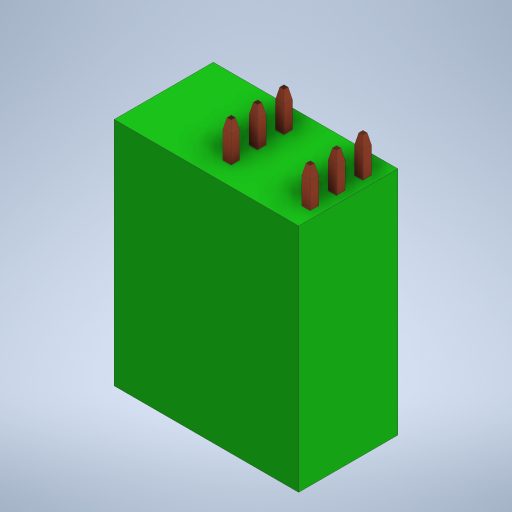
# Autodesk Inventor part: DB2ERH-2.5-2x3
Saved by Autodesk Inventor 2024 (Build 280153000, 153)
## iProperties
Created: 2023-05-22
Part Number: DB2ERH-2.5-2x3
Material: Generic
Document SubType Name: Modeling
Designer: torba
Density: 1 g/cm^3
Appearance: Default
Author: torba
Autodesk Inventor part; units mm, degrees
ref_plane "YZ Plane" through (0, 0, 0) normal (1, 0, 0) x (0, 1, 0)
ref_plane "XZ Plane" through (0, 0, 0) normal (0, 1, 0) x (-1, 0, 0)
ref_plane "XY Plane" through (0, 0, 0) normal (0, 0, 1) x (1, 0, 0)
sketch "Sketch1" plane through (0, 0, 0) normal (0, 1, 0) x (-1, 0, 0)
  line L0 (-0.4, 0.4) -> (0.4, 0.4)
  line L1 (0.4, 0.4) -> (0.4, -0.4)
  line L2 (0.4, -0.4) -> (-0.4, -0.4)
  line L3 (-0.4, -0.4) -> (-0.4, 0.4)
  line L4 (-0.4, 0.4) -> (0.4, -0.4) construction
  line L5 (0.4, 0.4) -> (-0.4, -0.4) construction
  line L6 (-0.4, -2.1) -> (0.4, -2.1)
  line L7 (0.4, -2.1) -> (0.4, -2.9)
  line L8 (0.4, -2.9) -> (-0.4, -2.9)
  line L9 (-0.4, -2.9) -> (-0.4, -2.1)
  line L10 (-0.4, -2.1) -> (0.4, -2.9) construction
  line L11 (0.4, -2.1) -> (-0.4, -2.9) construction
  line L12 (-0.4, -4.6) -> (0.4, -4.6)
  line L13 (0.4, -4.6) -> (0.4, -5.4)
  line L14 (0.4, -5.4) -> (-0.4, -5.4)
  line L15 (-0.4, -5.4) -> (-0.4, -4.6)
  line L16 (-0.4, -4.6) -> (0.4, -5.4) construction
  line L17 (0.4, -4.6) -> (-0.4, -5.4) construction
  line L18 (-7.9, 0.4) -> (-7.1, 0.4)
  line L19 (-7.1, 0.4) -> (-7.1, -0.4)
  line L20 (-7.1, -0.4) -> (-7.9, -0.4)
  line L21 (-7.9, -0.4) -> (-7.9, 0.4)
  line L22 (-7.9, 0.4) -> (-7.1, -0.4) construction
  line L23 (-7.1, 0.4) -> (-7.9, -0.4) construction
  line L24 (-7.9, -2.1) -> (-7.1, -2.1)
  line L25 (-7.1, -2.1) -> (-7.1, -2.9)
  line L26 (-7.1, -2.9) -> (-7.9, -2.9)
  line L27 (-7.9, -2.9) -> (-7.9, -2.1)
  line L28 (-7.9, -2.1) -> (-7.1, -2.9) construction
  line L29 (-7.1, -2.1) -> (-7.9, -2.9) construction
  line L30 (-7.9, -4.6) -> (-7.1, -4.6)
  line L31 (-7.1, -4.6) -> (-7.1, -5.4)
  line L32 (-7.1, -5.4) -> (-7.9, -5.4)
  line L33 (-7.9, -5.4) -> (-7.9, -4.6)
  line L34 (-7.9, -4.6) -> (-7.1, -5.4) construction
  line L35 (-7.1, -4.6) -> (-7.9, -5.4) construction
  line L36 (8.9, 2.2) -> (-8.6, 2.2)
  line L37 (-8.6, 2.2) -> (-8.6, -7.2)
  line L38 (-8.6, -7.2) -> (8.9, -7.2)
  line L39 (8.9, -7.2) -> (8.9, 2.2)
  point P0 (0, 0)
  point P1 (0, -2.5)
  point P2 (0, -5)
  point P3 (-7.5, 0)
  point P4 (-7.5, -2.5)
  point P5 (-7.5, -5)
  point P6 (0, -5)
  dimension "d0" = 0.8
  dimension "d1" = 0.8
  dimension "d4" = 2.5
  dimension "d7" = 7.5
  dimension "d10" = 17.5
  dimension "d11" = 9.4
  dimension "d12" = 2.2
  dimension "d13" = 2.2
  dimension "d14" = 8.9
  dimension "d48" = 8.2
  dimension "d49" = 11.85
  dimension "d37" = 0.8
  dimension "d38" = 0.8
  dimension "d39" = 4.2
  dimension "d42" = 2.5
  dimension "d45" = 13.8
  constraints: 80 end point, 4 parallel, 3 horizontal, 3 midpoint, 2 collinear, 2 perpendicular, 1 vertical, 53 other
  measures "d0" distance of L0.end L1.end
  measures "d1" distance of L1.end L2.end
  measures "d4" distance of L0.start L6.start
  measures "d7" distance of L0.start L18.start
  measures "d10" distance of L37.end L38.end
  measures "d11" distance of L38.end L36.start
  measures "d12" distance from line of L36 point (0, 0)
  measures "d13" distance from line of L38 point (0, -5)
  measures "d14" distance from line of L39 point (0, 0)
extrude "Extrusion1" add sketch "Sketch1" along normal blind 3.5 contours L0 L1 L2 L3 | L6 L7 L8 L9 | L12 L13 L14 L15 | L18 L19 L20 L21 | L24 L25 L26 L27 | L30 L31 L32 L33
chamfer "Chamfer1" distance 0.2 distance2 1 4 edges at (0.4, 3.5, 0) (0, 3.5, -0.4) (-0.4, 3.5, 0) (0, 3.5, 0.4) measured on face at (0.1333, 3.5, 0.1333)
chamfer "Chamfer2" distance 0.2 distance2 1 4 edges at (0, 3.5, -2.1) (-0.4, 3.5, -2.5) (0, 3.5, -2.9) (0.4, 3.5, -2.5) measured on face at (0.1333, 3.5, -2.3667)
chamfer "Chamfer3" distance 0.2 distance2 1 4 edges at (0, 3.5, -4.6) (-0.4, 3.5, -5) (0, 3.5, -5.4) (0.4, 3.5, -5) measured on face at (0.1333, 3.5, -4.8667)
chamfer "Chamfer4" distance 0.2 distance2 1 4 edges at (7.1, 3.5, 0) (7.5, 3.5, 0.4) (7.9, 3.5, 0) (7.5, 3.5, -0.4) measured on face at (7.6333, 3.5, 0.1333)
chamfer "Chamfer5" distance 0.2 distance2 1 4 edges at (7.5, 3.5, -2.1) (7.1, 3.5, -2.5) (7.5, 3.5, -2.9) (7.9, 3.5, -2.5) measured on face at (7.6333, 3.5, -2.3667)
chamfer "Chamfer6" distance 0.2 distance2 1 4 edges at (7.1, 3.5, -5) (7.5, 3.5, -4.6) (7.5, 3.5, -5.4) (7.9, 3.5, -5) measured on face at (7.6333, 3.5, -4.8667)
extrude "Extrusion2" add sketch "Sketch1" against normal blind 21.9 separate body contours L0 L1 L2 L3 | L6 L7 L8 L9 | L12 L13 L14 L15 | L18 L19 L20 L21 | L24 L25 L26 L27 | L30 L31 L32 L33 | L39 L38 L37 L36
